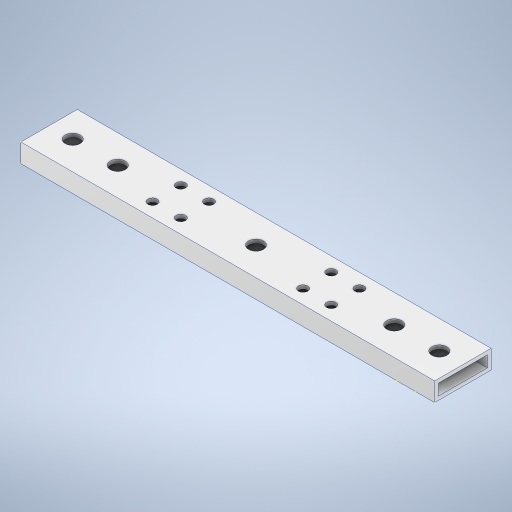
# Autodesk Inventor part: short_frame
Saved by Autodesk Inventor 2023 (Build 270158000, 158)
## iProperties
Created: 2022-12-19
Part Number: short_frame
Material: Aluminum 6061
Document SubType Name: Modeling
Designer: LAB-505
Density: 2.7 g/cm^3
Appearance: Aluminum - Flat
Mass: 81.1249 g
Surface Area: 314.401 cm^2
Volume: 30.0463 cm^3
Author: LAB-505
Autodesk Inventor part; units mm, degrees
ref_plane "YZ Plane" through (0, 0, 0) normal (1, 0, 0) x (0, 1, 0)
ref_plane "XZ Plane" through (0, 0, 0) normal (0, 1, 0) x (-1, 0, 0)
ref_plane "XY Plane" through (0, 0, 0) normal (0, 0, 1) x (1, 0, 0)
sketch "Sketch1" plane through (0, 0, 0) normal (1, 0, 0) x (0, 1, 0)
  point P0 (0, 0)
sketch "Sketch2" plane through (0, 0, 0) normal (1, 0, 0) x (0, 1, 0)
  point P0 (0, 0)
sketch "Sketch3" plane through (0, 0, 0) normal (1, 0, 0) x (0, 1, 0)
  line L0 (0, 0) -> (10, 0)
  line L1 (10, 0) -> (10, -30)
  line L2 (10, -30) -> (0, -30)
  line L3 (0, -30) -> (0, 0)
  line L4 (9, -29) -> (1, -29)
  line L5 (1, -29) -> (1, -1)
  line L6 (1, -1) -> (9, -1)
  line L7 (9, -1) -> (9, -29)
  dimension "d0" = 10
  dimension "d1" = 30
  dimension "d2" = 8
  dimension "d3" = 28
  constraints: 16 end point, 4 parallel, 2 horizontal, 2 perpendicular
  measures "d0" distance of L1.end L2.end
  measures "d1" distance of L0.end L1.end
  measures "d2" distance of L5.end L6.end
  measures "d3" distance of L4.end L5.end
extrude "Extrusion1" add sketch "Sketch3" along normal blind 200 contours L0 L1 L2 L3 | L4 L5 L6 L7
sketch "Sketch4" plane through (200, 0, 0) normal (1, 0, 0) x (0, 0, -1)
  line L0 (29, 9) -> (1, 9)
  line L1 (1, 9) -> (1, 1)
  line L2 (1, 1) -> (29, 1)
  line L3 (29, 1) -> (29, 9)
  point P0 (0, 0)
  dimension "d6" = 28
  dimension "d7" = 8
  constraints: 8 end point, 2 parallel, 1 horizontal, 1 perpendicular
  measures "d6" distance of L2.end L1.end
  measures "d7" distance of L1.end L0.end
extrude "Extrusion2" cut sketch "Sketch4" against normal blind 303.2375
sketch "Sketch5" plane through (0, 10, 0) normal (0, 1, 0) x (1, 0, 0)
  point P0 (0, 0)
sketch "Sketch6" plane through (200, 0, 0) normal (1, 0, 0) x (0, 0, -1)
  point P0 (0, 0)
sketch "Sketch7" plane through (200, 0, 0) normal (1, 0, 0) x (0, 0, -1)
  line L0 (0, 0) -> (30, 0) projected
  line L1 (30, 10) -> (0, 10) projected
  line L2 (30, 0) -> (0, 0)
  line L3 (0, 0) -> (0, 10)
  line L4 (0, 10) -> (30, 10)
  line L5 (30, 10) -> (30, 0)
  constraints: 8 end point, 2 parallel, 1 horizontal, 1 perpendicular
extrude "Extrusion3" add sketch "Sketch7" along normal blind 20
sketch "Sketch8" plane through (0, 0, 0) normal (-1, 0, 0) x (0, 0, 1)
  line L0 (-29, 9) -> (-1, 9)
  line L1 (-1, 9) -> (-1, 1)
  line L2 (-1, 1) -> (-29, 1)
  line L3 (-29, 1) -> (-29, 9)
  point P0 (0, 0)
  constraints: 8 end point, 2 parallel, 1 horizontal, 1 perpendicular
sketch "Sketch9" plane through (220, 0, 0) normal (1, 0, 0) x (0, 0, -1)
  line L0 (1, 1) -> (29, 1)
  line L1 (29, 1) -> (29, 9)
  line L2 (29, 9) -> (1, 9)
  line L3 (1, 9) -> (1, 1)
  point P0 (0, 0)
  constraints: 8 end point, 2 parallel, 1 horizontal, 1 perpendicular
extrude "Extrusion4" cut sketch "Sketch9" against normal blind 750.25
sketch "Sketch10" plane through (0, 10, 0) normal (0, 1, 0) x (1, 0, 0)
  circle A0 centre (22.5, 15) radius 4
  circle A1 centre (46.5, 15) radius 4
  point P0 (0, 0)
  dimension "d14" = 8
  dimension "d15" = 8
  constraints: 2 centre point
  measures "d14" diameter of A0
  measures "d15" diameter of A1
extrude "Extrusion5" cut sketch "Sketch10" against normal blind 63.025
sketch "Sketch11" plane through (0, 10, 0) normal (0, 1, 0) x (1, 0, 0)
  circle A0 centre (173.5, 15) radius 4
  circle A1 centre (197.5, 15) radius 4
  point P0 (0, 0)
  dimension "d18" = 8
  dimension "d19" = 8
  constraints: 2 centre point
  measures "d18" diameter of A0
  measures "d19" diameter of A1
extrude "Extrusion6" cut sketch "Sketch11" against normal blind 120.175
sketch "Sketch12" plane through (0, 10, 0) normal (0, 1, 0) x (1, 0, 0)
  line L0 (0, 30) -> (220, 30) projected
  line L1 (0, 0) -> (220, 0) projected
  line L2 (0, 30) -> (10, 30)
  line L3 (10, 30) -> (10, 0)
  line L4 (10, 0) -> (0, 0)
  line L5 (0, 0) -> (0, 30)
  dimension "d22" = 10
  constraints: 8 end point, 2 parallel, 1 horizontal, 1 perpendicular, 1 point on line
  measures "d22" distance of L3.end L4.end
extrude "Extrusion7" cut sketch "Sketch12" against normal blind 98.9
sketch "Sketch13" plane through (220, 10, 0) normal (0, 1, 0) x (1, 0, 0)
  line L0 (-210, 30) -> (0, 30) projected
  line L1 (0, 0) -> (-10, 0)
  line L2 (-10, 0) -> (-10, 30)
  line L3 (-10, 30) -> (0, 30)
  line L4 (0, 30) -> (0, 0)
  point P0 (-220, 0)
  dimension "d25" = 10
  constraints: 8 end point, 2 parallel, 1 horizontal, 1 perpendicular, 1 point on line
  measures "d25" distance of L2.end L3.end
extrude "Extrusion8" cut sketch "Sketch13" against normal blind 67.7875
sketch "Sketch14" plane through (10, 10, 0) normal (0, 1, 0) x (1, 0, 0)
  circle A0 centre (52.5, 7.5) radius 2.5
  circle A1 centre (52.5, 22.5) radius 2.5
  point P0 (-10, 0)
  dimension "d28" = 5
  dimension "d29" = 5
  constraints: 2 centre point
  measures "d28" diameter of A0
  measures "d29" diameter of A1
sketch "Sketch15" plane through (10, 10, 0) normal (0, 1, 0) x (1, 0, 0)
  circle A0 centre (67.5, 22.5) radius 2.5
  circle A1 centre (67.5, 7.5) radius 2.5
  point P0 (-10, 0)
  dimension "d30" = 5
  dimension "d31" = 5
  constraints: 2 centre point
  measures "d30" diameter of A0
  measures "d31" diameter of A1
extrude "Extrusion9" cut sketch "Sketch14" against normal blind 97.95
extrude "Extrusion10" cut sketch "Sketch15" against normal blind 108.425
sketch "Sketch16" plane through (10, 10, 0) normal (0, 1, 0) x (1, 0, 0)
  circle A0 centre (147.5, 22.5) radius 2.5
  circle A1 centre (132.5, 22.5) radius 2.5
  circle A2 centre (132.5, 7.5) radius 2.5
  circle A3 centre (147.5, 7.5) radius 2.5
  point P0 (-10, 0)
  dimension "d36" = 5
  dimension "d37" = 5
  dimension "d38" = 5
  dimension "d39" = 5
  constraints: 4 centre point
  measures "d36" diameter of A0
  measures "d37" diameter of A1
  measures "d38" diameter of A2
  measures "d39" diameter of A3
extrude "Extrusion11" cut sketch "Sketch16" against normal blind 59.85
sketch "Sketch17" plane through (10, 10, 0) normal (0, 1, 0) x (1, 0, 0)
  circle A0 centre (100, 15) radius 4
  point P0 (-10, 0)
  dimension "d42" = 8
  constraints: 1 centre point
  measures "d42" diameter of A0
extrude "Extrusion12" cut sketch "Sketch17" against normal blind 53.5
sketch "Sketch20" plane through (10, 10, -30) normal (-1, 0, 0) x (0, 0, 1)
  line L0 (30, -10) -> (0, -10) projected
  line L1 (30, 0) -> (0, 0) projected
  line L2 (30, -10) -> (0, -10)
  line L3 (0, -10) -> (0, 0)
  line L4 (0, 0) -> (30, 0)
  line L5 (30, 0) -> (30, -10)
  line L6 (29, -9) -> (1, -9) projected
  line L7 (29, -1) -> (1, -1) projected
  line L8 (29, -9) -> (1, -9)
  line L9 (1, -9) -> (1, -1)
  line L10 (1, -1) -> (29, -1)
  line L11 (29, -1) -> (29, -9)
  constraints: 16 end point, 4 parallel, 2 horizontal, 2 perpendicular
extrude "Extrusion13" add sketch "Sketch20" along normal blind 10 contours L0 L3 L1 L5 | L6 L9 L7 L11
extrude "Extrusion14" cut sketch "Sketch8" against normal blind 34.45
sketch "Sketch21" plane through (210, 10, 0) normal (1, 0, 0) x (0, 0, -1)
  line L0 (30, -10) -> (0, -10) projected
  line L1 (0, 0) -> (30, 0)
  line L2 (30, 0) -> (30, -10)
  line L3 (30, -10) -> (0, -10)
  line L4 (0, -10) -> (0, 0)
  line L5 (29, -1) -> (1, -1) projected
  line L6 (1, -9) -> (29, -9) projected
  line L7 (1, -1) -> (29, -1)
  line L8 (29, -1) -> (29, -9)
  line L9 (29, -9) -> (1, -9)
  line L10 (1, -9) -> (1, -1)
  constraints: 16 end point, 4 parallel, 2 horizontal, 2 perpendicular
extrude "Extrusion15" add sketch "Sketch21" along normal blind 10 contours L0 L4 L1 L2 | L8 L6 L10 L5
sketch "Sketch22" plane through (220, 10, 0) normal (1, 0, 0) x (0, 0, -1)
  point P0 (0, -10)
sketch "Sketch23" plane through (220, 10, 0) normal (1, 0, 0) x (0, 0, -1)
  point P0 (0, -10)
sketch "Sketch24" plane through (0, 10, -30) normal (-1, 0, 0) x (0, 0, 1)
  line L0 (2, -2) -> (28, -2)
  line L1 (28, -2) -> (28, -8)
  line L2 (28, -8) -> (2, -8)
  line L3 (2, -8) -> (2, -2)
  point P0 (30, -10)
  dimension "d51" = 26
  dimension "d52" = 6
  constraints: 8 end point, 2 parallel, 1 horizontal, 1 perpendicular
  measures "d51" distance of L1.end L2.end
  measures "d52" distance of L0.end L1.end
extrude "Extrusion16" add sketch "Sketch24" against normal blind 220
sketch "Sketch25" plane through (220, 10, 0) normal (1, 0, 0) x (0, 0, -1)
  line L0 (2, -8) -> (2, -2) projected
  line L1 (28, -2) -> (28, -8) projected
  line L2 (2, -8) -> (28, -8)
  line L3 (28, -8) -> (28, -2)
  line L4 (28, -2) -> (2, -2)
  line L5 (2, -2) -> (2, -8)
  point P0 (0, -10)
  constraints: 8 end point, 2 parallel, 1 horizontal, 1 perpendicular
extrude "Extrusion17" cut sketch "Sketch25" against normal blind 351.5
sketch "Sketch26" plane through (210, 10, 0) normal (-1, 0, 0) x (0, 0, 1)
  point P0 (0, -10)
sketch "Sketch27" plane through (0, 10, -30) normal (-1, 0, 0) x (0, 0, 1)
  line L0 (2, -2) -> (2, -8) projected
  line L1 (2, -8) -> (28, -8) projected
  line L2 (2, -2) -> (28, -2)
  line L3 (28, -2) -> (28, -8)
  line L4 (28, -8) -> (2, -8)
  line L5 (2, -8) -> (2, -2)
  line L6 (29, -1) -> (29, -9) projected
  line L7 (29, -9) -> (0.9924, -9)
  line L8 (0.9924, -9) -> (0.9924, -1)
  line L9 (0.9924, -1) -> (29, -1)
  line L10 (29, -1) -> (29, -9)
  point P0 (30, -10)
  constraints: 16 end point, 4 parallel, 2 horizontal, 2 perpendicular
extrude "Extrusion18" cut sketch "Sketch27" against normal blind 220
sketch "Sketch28" plane through (220, 10, 0) normal (1, 0, 0) x (0, 0, -1)
  line L0 (2, -8) -> (28, -8)
  line L1 (28, -8) -> (28, -2)
  line L2 (28, -2) -> (2, -2)
  line L3 (2, -2) -> (2, -8)
  line L4 (29.0076, -1) -> (1, -1) projected
  line L5 (1, -9) -> (29.0076, -9) projected
  line L6 (1, -1) -> (29.0076, -1)
  line L7 (29.0076, -1) -> (29.0076, -9)
  line L8 (29.0076, -9) -> (1, -9)
  line L9 (1, -9) -> (1, -1)
  point P0 (0, -10)
  dimension "d59" = 26
  dimension "d60" = 6
  constraints: 16 end point, 4 parallel, 2 horizontal, 2 perpendicular
  measures "d59" distance of L2.end L1.end
  measures "d60" distance of L1.end L0.end
extrude "Extrusion19" add sketch "Sketch28" against normal blind 220
sketch "Sketch29" plane through (0, 10, 0) normal (0, 1, 0) x (1, 0, 0)
  circle A0 centre (12.5, 15) radius 4
  point P0 (0, 0)
  dimension "d63" = 8
  constraints: 1 centre point
  measures "d63" diameter of A0
sketch "Sketch30" plane through (0, 10, 0) normal (0, 1, 0) x (1, 0, 0)
  circle A0 centre (36.5, 15) radius 4
  point P0 (0, 0)
  dimension "d64" = 8
  constraints: 1 centre point
  measures "d64" diameter of A0
extrude "Extrusion20" cut sketch "Sketch30" against normal blind 143.5375
extrude "Extrusion21" cut sketch "Sketch29" against normal blind 377.1625
sketch "Sketch31" plane through (22.5, 9, -15) normal (0, 1, 0) x (1, 0, 0)
  circle A0 centre (0, 0) radius 4
  circle A1 centre (24, 0) radius 4
  point P0 (-22.5, -15)
  constraints: 2 centre point
extrude "Extrusion22" cut sketch "Sketch31" against normal blind 135.6
sketch "Sketch32" plane through (0, 10, 0) normal (0, 1, 0) x (1, 0, 0)
  circle A0 centre (22.5, 15) radius 4 projected
  circle A1 centre (22.5, 15) radius 4
  circle A2 centre (46.5, 15) radius 4 projected
  circle A3 centre (46.5, 15) radius 4
  point P0 (0, 0)
  constraints: 2 centre point, 2 coincident
extrude "Extrusion23" add sketch "Sketch32" against normal blind 2
sketch "Sketch33" plane through (0, 0, -30) normal (0, -1, 0) x (1, 0, 0)
  circle A0 centre (46.5, 14.9969) radius 4
  circle A1 centre (22.5, 14.9969) radius 4
  point P0 (0, 30)
  dimension "d73" = 8
  dimension "d74" = 8
  constraints: 2 centre point
  measures "d73" diameter of A0
  measures "d74" diameter of A1
extrude "Extrusion24" add sketch "Sketch33" against normal blind 2
sketch "Sketch36" plane through (0, 10, 0) normal (0, 1, 0) x (1, 0, 0)
  circle A0 centre (207.5, 15) radius 4
  circle A1 centre (183.5, 15) radius 4
  point P0 (0, 0)
  dimension "d77" = 8
  dimension "d78" = 8
  constraints: 2 centre point
  measures "d77" diameter of A0
  measures "d78" diameter of A1
extrude "Extrusion25" cut sketch "Sketch36" against normal blind 72.6125
sketch "Sketch37" plane through (0, 10, 0) normal (0, 1, 0) x (1, 0, 0)
  circle A0 centre (197.5, 15) radius 4 projected
  circle A1 centre (197.5, 15) radius 4
  circle A2 centre (173.5, 15) radius 4 projected
  circle A3 centre (173.5, 15) radius 4
  point P0 (0, 0)
  constraints: 2 centre point, 2 coincident
extrude "Extrusion26" add sketch "Sketch37" against normal blind 2
sketch "Sketch38" plane through (0, 0, -30) normal (0, -1, 0) x (1, 0, 0)
  circle A0 centre (173.5, 15) radius 4 projected
  circle A1 centre (173.5, 15) radius 4
  circle A2 centre (197.5, 15) radius 4 projected
  circle A3 centre (197.5, 15) radius 4
  point P0 (0, 30)
  constraints: 2 centre point, 2 coincident
extrude "Extrusion27" add sketch "Sketch38" against normal blind 2
sketch "Sketch39" plane through (0, 0, -30) normal (0, -1, 0) x (1, 0, 0)
  circle A0 centre (62.5, 22.5) radius 2.5 projected
  circle A1 centre (62.5, 22.5) radius 2.5
  circle A2 centre (77.5, 22.5) radius 2.5 projected
  circle A3 centre (77.5, 22.5) radius 2.5
  circle A4 centre (77.5, 7.5) radius 2.5 projected
  circle A5 centre (77.5, 7.5) radius 2.5
  circle A6 centre (62.5, 7.5) radius 2.5 projected
  circle A7 centre (62.5, 7.5) radius 2.5
  circle A8 centre (142.5, 22.5) radius 2.5 projected
  circle A9 centre (142.5, 22.5) radius 2.5
  circle A10 centre (157.5, 22.5) radius 2.5 projected
  circle A11 centre (157.5, 22.5) radius 2.5
  circle A12 centre (157.5, 7.5) radius 2.5 projected
  circle A13 centre (157.5, 7.5) radius 2.5
  circle A14 centre (142.5, 7.5) radius 2.5 projected
  circle A15 centre (142.5, 7.5) radius 2.5
  circle A16 centre (110, 15) radius 4 projected
  circle A17 centre (110, 15) radius 4
  point P0 (0, 30)
  constraints: 9 centre point, 9 coincident
extrude "Extrusion28" cut sketch "Sketch39" against normal blind 68.675
body "Solid1"
